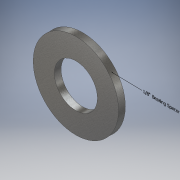
# Autodesk Inventor part: 1-8inch_BearingSpacer_Piece1
Saved by Autodesk Inventor 2018 (Build 220112000, 112)
## iProperties
Created: 2018-01-22
Part Number: 1-8inch_BearingSpacer_Piece1
Material: Generic
Document SubType Name: Modeling
Designer: Olivier
Density: 1 g/cm^3
Appearance: Default
Author: Olivier
Autodesk Inventor part; units mm, degrees
ref_plane "YZ Plane" through (0, 0, 0) normal (1, 0, 0) x (0, 1, 0)
ref_plane "XZ Plane" through (0, 0, 0) normal (0, 1, 0) x (-1, 0, 0)
ref_plane "XY Plane" through (0, 0, 0) normal (0, 0, 1) x (1, 0, 0)
sketch "Sketch1" plane through (0, 0, 0) normal (0, 0, 1) x (1, 0, 0)
  circle A0 centre (0, 0) radius 20
  circle A1 centre (0, 0) radius 10.1
  circle A2 centre (0, 0) radius 20
  circle A3 centre (0, 0) radius 10.1
  dimension "d2" = 0.5822
  dimension "d3" = 0.1082
  constraints: 4 centre point
extrude "Extrusion1" add sketch "Sketch1" along normal blind 3.175
body "Solid1"
